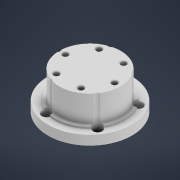
# Autodesk Inventor part: OutputShaft2
Saved by Autodesk Inventor 2022 (Build 260153000, 153)
## iProperties
Created: 2022-10-09
Part Number: OutputShaft2
Material: Ogólny
Document SubType Name: Modeling
Designer: MicnedSQ
Density: 1 g/cm^3
Appearance: Domyślna
Author: MicnedSQ
## iProperties of the stored document OutputShaft2_3DPrint.ipt
Created: 2022-10-23
Part Number: OutputShaft2_3DPrint
Material: Generic
Document SubType Name: Modeling
Designer: MicnedSQ
Density: 1 g/cm^3
Appearance: Default
Author: MicnedSQ
Autodesk Inventor part; units mm, degrees
ref_plane "YZ Plane" through (0, 0, 0) normal (1, 0, 0) x (0, 1, 0)
ref_plane "XZ Plane" through (0, 0, 0) normal (0, 1, 0) x (-1, 0, 0)
ref_plane "XY Plane" through (0, 0, 0) normal (0, 0, 1) x (1, 0, 0)
sketch "Szkic1" plane through (0, 0, 0) normal (0, 1, 0) x (-1, 0, 0)
  circle A0 centre (0, 0) radius 27.25
  dimension "d0" = 54.5
  constraints: 1 centre point, 1 coincident
  measures "d0" diameter of A0
extrude "Wyciągnięcie proste1" add sketch "Szkic1" along normal blind 6
sketch "Szkic2" plane through (0, 6, 0) normal (0, 1, 0) x (1, 0, 0)
  circle A0 centre (0, 0) radius 22.5
  dimension "d3" = 45
  constraints: 1 centre point, 1 coincident
  measures "d3" diameter of A0
extrude "Wyciągnięcie proste2" add sketch "Szkic2" along normal blind 1
sketch "Szkic3" plane through (0, 7, 0) normal (0, 1, 0) x (1, 0, 0)
  circle A0 centre (0, 0) radius 20
  dimension "d6" = 40
  constraints: 1 centre point, 1 coincident
  measures "d6" diameter of A0
extrude "Wyciągnięcie proste3" add sketch "Szkic3" along normal blind 17
sketch "Szkic4" plane through (0, 6, 0) normal (0, 1, 0) x (1, 0, 0)
  circle A0 centre (-22.5, 0) radius 3
  point P0 (0, 0)
  dimension "d9" = 6
  dimension "d10" = 22.5
  constraints: 1 centre point
  measures "d9" diameter of A0
  measures "d10" distance of point (0, 0) A0.centre
extrude "Wyciągnięcie proste4" cut sketch "Szkic4" along normal blind 18 and the other way blind 4
sketch "Szkic5" plane through (-22.5, 2, 0) normal (0, 1, 0) x (1, 0, 0)
  circle A0 centre (0, 0) radius 1.75
  point P0 (22.5, 0)
  dimension "d15" = 3.5
  constraints: 1 centre point
  measures "d15" diameter of A0
extrude "Wyciągnięcie proste5" cut sketch "Szkic5" against normal up to surface (2 mm away)
pattern_circular "Szyk kołowy1" count 5 over 360 about axis through (0, 0, 0) along (0, 1, 0) of "Wyciągnięcie proste4", "Wyciągnięcie proste5"
sketch "Szkic6" plane through (0, 0, 0) normal (0, -1, 0) x (1, 0, 0)
  circle A0 centre (0, 0) radius 16.15
  dimension "d21" = 32.3
  constraints: 1 centre point, 1 coincident
  measures "d21" diameter of A0
extrude "Wyciągnięcie proste6" cut sketch "Szkic6" against normal blind 3
sketch "Szkic7" plane through (0, 3, 0) normal (0, -1, 0) x (1, 0, 0)
  circle A0 centre (0, 0) radius 14
  dimension "d24" = 28
  constraints: 1 centre point, 1 coincident
  measures "d24" diameter of A0
extrude "Wyciągnięcie proste7" cut sketch "Szkic7" against normal blind 5
sketch "Sketch8" plane through (0, 24, 0) normal (0, 1, 0) x (1, 0, 0)
  circle A0 centre (0, 0) radius 16.15 projected
  circle A1 centre (16, 0) radius 1.85
  dimension "d27" = 3.7
  dimension "d28" = 16
  constraints: 1 centre point
  measures "d27" diameter of A1
  measures "d28" distance of point (0, 0) A1.centre
extrude "Extrusion8" cut sketch "Sketch8" against normal blind 12 contours A0 A1 | A0 A1 picked at (15.5207, 0.4277) picked at (16.6977, 0.3411)
pattern_circular "Circular Pattern2" count 6 over 360 about axis through (0, 7, 0) along (0, 1, 0) of "Extrusion8"
